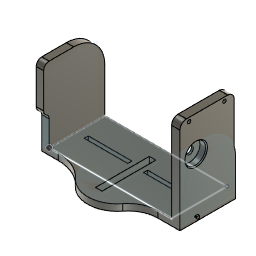
Cradle (Autodesk Fusion 360 design; units mm, degrees)
Autodesk Fusion 360 part; units mm, degrees
note: some values were not read from the file. Chosen so that the rebuilt part matches the saved one: which face or edge a step refers to; which pieces of a blend or face edit are solid. Set by a fixed rule: which sketch regions a step uses.
sketch "Szkic1" plane through (0, 0, 0) normal (0, 0, 1) x (1, 0, 0)
  line L0 (0, 0) -> (149, 0)
  line L1 (149, 0) -> (149, -85)
  line L2 (149, -85) -> (0, -85)
  line L3 (0, -85) -> (0, 0)
  line L4 (0, -85) -> (55, -85)
  line L5 (55, -85) -> (55, -60)
  line L6 (55, -60) -> (0, -60)
  line L7 (0, -60) -> (0, -85)
  line L8 (149, -85) -> (94, -85)
  line L9 (94, -85) -> (94, -60)
  line L10 (94, -60) -> (149, -60)
  line L11 (149, -60) -> (149, -85)
  dimension "d1" = 149
  dimension "d2" = 85
  dimension "d3" = 55
  dimension "d4" = 25
  dimension "d5" = 55
  dimension "d6" = 25
  constraint horizontal L0
  constraint vertical L1
  constraint horizontal L2
  constraint vertical L3
  constraint coincident L0.start L3.end
  constraint horizontal L4
  constraint vertical L5
  constraint horizontal L6
  constraint vertical L7
  constraint horizontal L8
  constraint vertical L9
  constraint horizontal L10
  constraint vertical L11
  measures "d1" distance of L0.start L0.end
  measures "d2" distance of L0.start L2.end
  measures "d3" distance of L2.end L4.end
  measures "d4" distance of L2.end L6.end
  measures "d5" distance of L1.end L8.end
  measures "d6" distance of L1.end L10.end
extrude "Wyciągnięcie proste1" add sketch "Szkic1" along normal blind 4 contours L0 L1 L2 L3 L5 L6 L9 L10
fillet "Zaokrąglenie1" radius 32 4 edges at (94, -60, 2) (94, -85, 2) (55, -85, 2) (55, -60, 2)
sketch "Szkic2" plane through (0, 0, 4) normal (0, 0, 1) x (-1, 0, 0)
  arc A0 (-49.1375, 72.4873) -> (-99.8528, 72.5) centre (-74.5, 52.9747) ccw
  arc A1 (-99.8625, 72.4873) -> (-99.8528, 72.5) centre (-125.225, 92) ccw
  arc A2 (-125.225, 60) -> (-99.8625, 72.4873) centre (-125.225, 92) ccw
  line L0 (-125.225, 60) -> (-149, 60)
  line L1 (-149, 60) -> (-149, 0)
  line L2 (-149, 0) -> (0, 0)
  line L3 (0, 0) -> (0, 60)
  line L4 (0, 60) -> (-23.775, 60)
  arc A3 (-49.1375, 72.4873) -> (-23.775, 60) centre (-23.775, 92) ccw
  line L5 (0, 0) -> (-8, 0)
  line L6 (-8, 0) -> (-8, 60)
  line L7 (-8, 60) -> (0, 60)
  line L8 (0, 60) -> (0, 0)
  line L9 (-149, 0) -> (-145, 0)
  line L10 (-145, 0) -> (-145, 60)
  line L11 (-145, 60) -> (-149, 60)
  line L12 (-149, 60) -> (-149, 0)
  constraint horizontal L5
  constraint vertical L6
  constraint horizontal L7
  constraint vertical L8
  constraint coincident L4 L6.end
  constraint coincident L2.end L3.start
  constraint horizontal L9
  constraint vertical L10
  constraint horizontal L11
  constraint vertical L12
  constraint coincident L0 L10.end
  constraint coincident L1.end L2.start
extrude "Wyciągnięcie proste2" add sketch "Szkic2" along normal blind 66 contours L2 L3 L4 L5 L6 L7 L8 | L0 L1 L2 L9 L10 L11 L12
sketch "Szkic3" plane through (0, 0, 0) normal (-1, 0, 0) x (0, -1, 0)
  line L0 (0, 0) -> (60, 0)
  line L1 (60, 0) -> (60, 70)
  line L2 (60, 70) -> (0, 70)
  line L3 (0, 70) -> (0, 0)
  circle A0 centre (42.5, 60) radius 4
  dimension "d15" = 8
  measures "d15" diameter of A0
extrude "Wyciągnięcie proste3" cut sketch "Szkic3" against normal blind 148 contours A0
extrude "Wyciągnięcie proste4" cut 1 faces at (148, -41.2702, 59.8013) along direction (1, 0, 0) blind 1
sketch "Szkic4" plane through (0, 0, 0) normal (-1, 0, 0) x (0, -1, 0)
  circle A0 centre (42.5, 60) radius 4
  line L0 (0, 0) -> (60, 0)
  line L1 (60, 0) -> (60, 70)
  line L2 (60, 70) -> (0, 70)
  line L3 (0, 70) -> (0, 0)
extrude "Wyciągnięcie proste5" add 1 faces at (5.3333, -40, 70) along direction (0, 0, 1) blind 15
sketch "Szkic5" plane through (0, -60, 0) normal (0, -1, 0) x (1, 0, 0)
  line L0 (23.775, 0) -> (23.775, 4)
  line L1 (23.775, 4) -> (8, 4)
  line L2 (8, 4) -> (8, 85)
  line L3 (8, 85) -> (0, 85)
  line L4 (0, 85) -> (0, 0)
  line L5 (0, 0) -> (23.775, 0)
  line L6 (0, 85) -> (8, 85)
  line L7 (8, 85) -> (8, 41)
  line L8 (8, 41) -> (0, 41)
  line L9 (0, 41) -> (0, 85)
  constraint horizontal L6
  constraint vertical L7
  constraint horizontal L8
  constraint vertical L9
  constraint coincident L2 L7.end
  constraint coincident L3.end L4.start
extrude "Wyciągnięcie proste6" add sketch "Szkic5" along normal blind 11 contours L2 L3 L4 L6 L7 L8 L9
sketch "Szkic6" plane through (0, 0, 0) normal (-1, 0, 0) x (0, -1, 0)
extrude "Wyciągnięcie proste7" add 1 faces at (5.3333, -63.6667, 41) along direction (0, 0, -1) blind 4
sketch "Szkic7" plane through (0, 0, 0) normal (-1, 0, 0) x (0, -1, 0)
  circle A0 centre (25.5, 77) radius 1.8
  circle A1 centre (59.5, 77) radius 1.8
  circle A2 centre (59.5, 43) radius 1.8
  circle A3 centre (25.5, 43) radius 1.8
  dimension "d28" = 3.6
  dimension "d29" = 3.6
  dimension "d30" = 3.6
  dimension "d31" = 3.6
  measures "d28" diameter of A0
  measures "d29" diameter of A1
  measures "d30" diameter of A2
  measures "d31" diameter of A3
extrude "Wyciągnięcie proste8" cut sketch "Szkic7" against normal blind 5.5
delete_face "Usuń powierzchnię1" 1 faces at (2.6667, -46.4801, 59.6017)
extrude "Wyciągnięcie proste9" cut 1 faces at (2.6667, -71, 53) along direction (0, 1, 0) blind 5
fillet "Zaokrąglenie2" radius 6 3 edges at (4, -60, 37) (4, -66, 37) (4, -66, 85)
fillet "Zaokrąglenie3" radius 33.5 2 edges at (147, 0, 70) (4, 0, 85)
sketch "Szkic8" plane through (0, 0, 4) normal (0, 0, 1) x (-1, 0, 0)
  line L0 (-145, 60) -> (-145, 0)
  line L1 (-145, 0) -> (-8, 0)
  line L2 (-8, 0) -> (-8, 60)
  line L3 (-8, 60) -> (-23.775, 60)
  arc A0 (-49.1375, 72.4873) -> (-23.775, 60) centre (-23.775, 92) ccw
  arc A1 (-49.1375, 72.4873) -> (-99.8528, 72.5) centre (-74.5, 52.9747) ccw
  arc A2 (-99.8625, 72.4873) -> (-99.8528, 72.5) centre (-125.225, 92) ccw
  arc A3 (-125.225, 60) -> (-99.8625, 72.4873) centre (-125.225, 92) ccw
  line L4 (-125.225, 60) -> (-145, 60)
  line L5 (-73, 14) -> (-80, 14)
  line L6 (-80, 14) -> (-80, 72)
  line L7 (-80, 72) -> (-73, 72)
  line L8 (-73, 72) -> (-73, 14)
  line L9 (-18, 27.8) -> (-68, 27.8)
  line L10 (-68, 27.8) -> (-68, 32.2)
  line L11 (-68, 32.2) -> (-18, 32.2)
  line L12 (-18, 32.2) -> (-18, 27.8)
  line L13 (-85, 27.8) -> (-135, 27.8)
  line L14 (-135, 27.8) -> (-135, 32.2)
  line L15 (-135, 32.2) -> (-85, 32.2)
  line L16 (-85, 32.2) -> (-85, 27.8)
  constraint horizontal L5
  constraint vertical L6
  constraint horizontal L7
  constraint vertical L8
  constraint horizontal L9
  constraint vertical L10
  constraint horizontal L11
  constraint vertical L12
  constraint horizontal L13
  constraint vertical L14
  constraint horizontal L15
  constraint vertical L16
extrude "Wyciągnięcie proste10" cut sketch "Szkic8" against normal blind 5 contours L5 L6 L7 L8 | L9 L10 L11 L12 | L13 L14 L15 L16
sketch "Szkic9" plane through (149, 0, 0) normal (1, 0, 0) x (0, 1, 0)
  arc A0 (0, 36.5) -> (-33.5, 70) centre (-33.5, 36.5) ccw
  line L0 (-33.5, 70) -> (-60, 70)
  line L1 (-60, 70) -> (-60, 0)
  line L2 (-60, 0) -> (0, 0)
  line L3 (0, 0) -> (0, 36.5)
  circle A1 centre (-42.5, 60) radius 4
  line L4 (-42.5, 60) -> (-42.5, 0)
  line L5 (-42.5, 0) -> (-41, 0)
  line L6 (-41, 0) -> (-41, 3)
  line L7 (-41, 3) -> (-42.5, 3)
  line L8 (-42.5, 3) -> (-42.5, 0)
  line L9 (-42.5, 3) -> (-44, 3)
  line L10 (-44, 3) -> (-44, 0)
  line L11 (-44, 0) -> (-42.5, 0)
  line L12 (-42.5, 0) -> (-42.5, 3)
  constraint coincident A1.centre L4.start
  constraint coincident L2 L4.end
  constraint perpendicular L2 L4
  constraint horizontal L5
  constraint vertical L6
  constraint horizontal L7
  constraint vertical L8
  constraint horizontal L9
  constraint vertical L10
  constraint horizontal L11
  constraint vertical L12
extrude "Wyciągnięcie proste11" add sketch "Szkic9" along normal blind 2 contours L2 L4 L5 L6 L7 L8 L12 | L2 L4 L8 L9 L10 L11 L12
fillet "Zaokrąglenie4" radius 2.25 1 edges at (150, -44, 0)
sketch "Szkic10" plane through (149, 0, 0) normal (1, 0, 0) x (0, 1, 0)
  line L0 (-41, 3) -> (-41, 0)
  line L1 (-41, 0) -> (0, 0)
  line L2 (0, 0) -> (0, 36.5)
  arc A0 (0, 36.5) -> (-33.5, 70) centre (-33.5, 36.5) ccw
  line L3 (-33.5, 70) -> (-60, 70)
  line L4 (-60, 70) -> (-60, 0)
  line L5 (-60, 0) -> (-41.75, 0)
  arc A1 (-44, 2.25) -> (-41.75, 0) centre (-41.75, 2.25) ccw
  line L6 (-44, 2.25) -> (-44, 3)
  line L7 (-44, 3) -> (-41, 3)
  circle A2 centre (-42.5, 60) radius 4
sketch "Szkic11" plane through (0, 0, 70) normal (0, 0, 1) x (-1, 0, 0)
  line L0 (-149, 33.5) -> (-145, 33.5)
  line L1 (-145, 33.5) -> (-145, 60)
  line L2 (-145, 60) -> (-149, 60)
  line L3 (-149, 60) -> (-149, 33.5)
delete_face "Usuń powierzchnię2" 1 faces at (33.3846, -61.477, 2.6667)
sketch "Szkic12" plane through (0, -60, 0) normal (0, -1, 0) x (1, 0, 0)
  line L0 (0, 0) -> (43.2807, 0)
  line L1 (43.2807, 0) -> (43.2807, 4)
  line L2 (43.2807, 4) -> (8, 4)
  line L3 (8, 4) -> (8, 31)
  line L4 (8, 31) -> (0, 31)
  line L5 (0, 31) -> (0, 0)
extrude "Wyciągnięcie proste13" add 1 faces at (5.3333, -42.3333, 85) along direction (0, 0, 1) blind 25
fillet "Zaokrąglenie7" radius 5 2 edges at (4, -60, 110) (4, -33.5, 110)
sketch "Szkic14" plane through (0, 0, 0) normal (-1, 0, 0) x (0, -1, 0)
  arc A0 (38.5, 110) -> (33.5, 105) centre (38.5, 105) ccw
  line L0 (33.5, 105) -> (33.5, 85)
  arc A1 (33.5, 85) -> (0, 51.5) centre (33.5, 51.5) ccw
  line L1 (0, 51.5) -> (0, 0)
  line L2 (0, 0) -> (60, 0)
  line L3 (60, 0) -> (60, 31)
  arc A2 (63, 36.1962) -> (60, 31) centre (66, 31) ccw
  arc A3 (63, 36.1962) -> (66, 41.3923) centre (60, 41.3923) ccw
  line L4 (66, 41.3923) -> (66, 79)
  arc A4 (66, 79) -> (60, 85) centre (60, 79) ccw
  line L5 (60, 85) -> (60, 105)
  arc A5 (60, 105) -> (55, 110) centre (55, 105) ccw
  line L6 (55, 110) -> (38.5, 110)
  circle A6 centre (25.5, 77) radius 1.8
  circle A7 centre (25.5, 43) radius 1.8
  circle A8 centre (59.5, 77) radius 1.8
  circle A9 centre (59.5, 43) radius 1.8
  circle A10 centre (45, 100) radius 1.8
  dimension "d63" = 3.6
  measures "d63" diameter of A10
extrude "Wyciągnięcie proste14" cut sketch "Szkic14" against normal blind 5.2 contours A10
sketch "Szkic15" plane through (8, 0, 0) normal (1, 0, 0) x (0, 1, 0)
  arc A0 (-33.5, 105) -> (-38.5, 110) centre (-38.5, 105) ccw
  line L0 (-38.5, 110) -> (-55, 110)
  arc A1 (-55, 110) -> (-60, 105) centre (-55, 105) ccw
  line L1 (-60, 105) -> (-60, 85)
  arc A2 (-60, 85) -> (-66, 79) centre (-60, 79) ccw
  line L2 (-66, 79) -> (-66, 41.3923)
  arc A3 (-66, 41.3923) -> (-63, 36.1962) centre (-60, 41.3923) ccw
  arc A4 (-60, 31) -> (-63, 36.1962) centre (-66, 31) ccw
  line L3 (-60, 31) -> (-60, 4)
  line L4 (-60, 4) -> (0, 4)
  line L5 (0, 4) -> (0, 51.5)
  arc A5 (0, 51.5) -> (-33.5, 85) centre (-33.5, 51.5) ccw
  line L6 (-33.5, 85) -> (-33.5, 105)
  circle A6 centre (-54, 104) radius 1.8
  dimension "d66" = 3.6
  measures "d66" diameter of A6
extrude "Wyciągnięcie proste15" cut sketch "Szkic15" against normal blind 5.2 contours A6
sketch "Szkic16" plane through (5.5, 0, 0) normal (-1, 0, 0) x (0, -1, 0)
  circle A0 centre (25.5, 77) radius 1.8
extrude "Wyciągnięcie proste16" add 1 faces at (145, -33.87, 32.2001) along direction (-1, 0, 0) blind 5
sketch "Szkic17" plane through (149, 0, 0) normal (1, 0, 0) x (0, 1, 0)
  circle A0 centre (-42.5, 60) radius 11
  dimension "d71" = 22
  measures "d71" diameter of A0
extrude "Wyciągnięcie proste17" add sketch "Szkic11" 1 faces at (144.6667, -42.3333, 70) along normal blind 3
extrude "Wyciągnięcie proste18" cut sketch "Szkic17" against normal blind 7
sketch "Szkic18" plane through (0, 0, 4) normal (0, 0, 1) x (-1, 0, 0)
  line L0 (-68, 27.8) -> (-68, 32.2)
  line L1 (-68, 32.2) -> (-18, 32.2)
  line L2 (-18, 32.2) -> (-18, 27.8)
  line L3 (-18, 27.8) -> (-68, 27.8)
  line L4 (-135, 27.8) -> (-135, 32.2)
  line L5 (-135, 32.2) -> (-85, 32.2)
  line L6 (-85, 32.2) -> (-85, 27.8)
  line L7 (-85, 27.8) -> (-135, 27.8)
  line L8 (-80, 14) -> (-80, 72)
  line L9 (-80, 72) -> (-73, 72)
  line L10 (-73, 72) -> (-73, 14)
  line L11 (-73, 14) -> (-80, 14)
  line L12 (-140, 60) -> (-140, 0)
  line L13 (-140, 0) -> (-8, 0)
  line L14 (-8, 0) -> (-8, 60)
  line L15 (-8, 60) -> (-43.2807, 60)
  arc A0 (-43.2807, 60) -> (-99.8625, 72.4873) centre (-74.5, 52.9747) ccw
  arc A1 (-125.225, 60) -> (-99.8625, 72.4873) centre (-125.225, 92) ccw
  line L16 (-125.225, 60) -> (-140, 60)
  line L17 (-140, 0) -> (-8, 0)
  line L18 (-8, 0) -> (-8, 60)
  line L19 (-8, 60) -> (-140, 60)
  line L20 (-140, 60) -> (-140, 0)
  constraint horizontal L17
  constraint vertical L18
  constraint horizontal L19
  constraint vertical L20
  constraint coincident L14.end L15.start
  constraint coincident L12.end L13.start
sketch "Szkic20" plane through (0, 0, 4) normal (0, 0, 1) x (-1, 0, 0)
fillet "Zaokrąglenie9" radius 45 1 edges at (43.2807, -60, 2)
sketch "Szkic21" plane through (0, 0, 4) normal (0, 0, 1) x (1, 0, 0)
extrude "Wyciągnięcie proste20" add 1 faces at (80, -33.3333, 2.6667) along direction (-1, 0, 0) blind 3
extrude "Wyciągnięcie proste21" cut 1 faces at (73, -52.6667, 2.6667) along direction (-1, 0, 0) blind 3
extrude "Wyciągnięcie proste22" add 1 faces at (68, -29.2667, 2.6667) along direction (-1, 0, 0) blind 3
extrude "Wyciągnięcie proste23" cut 1 faces at (85, -30.7333, 2.6667) along direction (-1, 0, 0) blind 3
sketch "Szkic22" plane through (0, 0, 4) normal (0, 0, 1) x (-1, 0, 0)
extrude "Wyciągnięcie proste24" add 1 faces at (146, -33.5, 71) along direction (0, 1, 0) blind 32
extrude "Wyciągnięcie proste25" add 1 faces at (143, -22.8333, 70) along direction (0, 0, -1) blind 39
extrude "Wyciągnięcie proste26" add 1 faces at (143, -40.5, 73) along direction (0, 0, 1) blind 25
sketch "Szkic23" plane through (149, 0, 0) normal (1, 0, 0) x (0, 1, 0)
  line L0 (-1.5, 46.4121) -> (-1.5, 98)
  line L1 (-1.5, 98) -> (-60, 98)
  line L2 (-60, 98) -> (-60, 0)
  line L3 (-60, 0) -> (-41.75, 0)
  arc A0 (-44, 2.25) -> (-41.75, 0) centre (-41.75, 2.25) ccw
  line L4 (-44, 2.25) -> (-44, 3)
  line L5 (-44, 3) -> (-41, 3)
  line L6 (-41, 3) -> (-41, 0)
  line L7 (-41, 0) -> (0, 0)
  line L8 (0, 0) -> (0, 36.5)
  arc A1 (0, 36.5) -> (-1.5, 46.4121) centre (-33.5, 36.5) ccw
  line L9 (-33.5, 66.3246) -> (-33.5, 53.6754)
  circle A2 centre (-42.5, 60) radius 11.16
  arc A3 (-33.5, 66.3246) -> (-33.5, 53.6754) centre (-42.5, 60) ccw
  dimension "d103" = 22.32
  measures "d103" diameter of A2
extrude "Wyciągnięcie proste27" cut sketch "Szkic23" against normal blind 7 contours L9 A3 | A2
chamfer "Fazowanie2" distance 1 angle 45 1 edges at (149, -52.9048, 64.0356)
sketch "Szkic24" plane through (149, 0, 0) normal (1, 0, 0) x (0, 1, 0)
  line L0 (-1.5, 46.4121) -> (-1.5, 98)
  line L1 (-1.5, 98) -> (-60, 98)
  line L2 (-60, 98) -> (-60, 0)
  line L3 (-60, 0) -> (-41.75, 0)
  arc A0 (-44, 2.25) -> (-41.75, 0) centre (-41.75, 2.25) ccw
  line L4 (-44, 2.25) -> (-44, 3)
  line L5 (-44, 3) -> (-41, 3)
  line L6 (-41, 3) -> (-41, 0)
  line L7 (-41, 0) -> (0, 0)
  line L8 (0, 0) -> (0, 36.5)
  arc A1 (0, 36.5) -> (-1.5, 46.4121) centre (-33.5, 36.5) ccw
  circle A2 centre (-42.5, 60) radius 12.16
  circle A3 centre (-50, 94) radius 1.8
  circle A4 centre (-12, 94) radius 1.8
  dimension "d107" = 3.6
  dimension "d108" = 3.6
  measures "d107" diameter of A3
  measures "d108" diameter of A4
fillet "Zaokrąglenie10" radius 7 2 edges at (144.5, -60, 98) (144.5, -1.5, 98)
sketch "Szkic25" plane through (0, 0, 0) normal (-1, 0, 0) x (0, -1, 0)
  circle A0 centre (45, 100) radius 1.8
  arc A1 (38.5, 110) -> (33.5, 105) centre (38.5, 105) ccw
  line L0 (33.5, 105) -> (33.5, 85)
  arc A2 (33.5, 85) -> (0, 51.5) centre (33.5, 51.5) ccw
  line L1 (0, 51.5) -> (0, 0)
  line L2 (0, 0) -> (60, 0)
  line L3 (60, 0) -> (60, 31)
  arc A3 (63, 36.1962) -> (60, 31) centre (66, 31) ccw
  arc A4 (63, 36.1962) -> (66, 41.3923) centre (60, 41.3923) ccw
  line L4 (66, 41.3923) -> (66, 79)
  arc A5 (66, 79) -> (60, 85) centre (60, 79) ccw
  line L5 (60, 85) -> (60, 105)
  arc A6 (60, 105) -> (55, 110) centre (55, 105) ccw
  line L6 (55, 110) -> (38.5, 110)
  circle A7 centre (25.5, 77) radius 1.8
  circle A8 centre (25.5, 43) radius 1.8
  circle A9 centre (59.5, 77) radius 1.8
  circle A10 centre (59.5, 43) radius 1.8
  line L7 (33.5, 85) -> (60, 85)
  line L8 (60, 85) -> (60, 110)
  line L9 (60, 110) -> (33.5, 110)
  line L10 (33.5, 110) -> (33.5, 85)
  constraint horizontal L7
  constraint vertical L8
  constraint horizontal L9
  constraint vertical L10
  constraint coincident L0.end A2.start
extrude "Wyciągnięcie proste28" cut sketch "Szkic25" against normal blind 10 contours A0 | A1 L0 L5 A6 L6 L7 L8 L9 L10
extrude "Wyciągnięcie proste29" cut sketch "Szkic24" against normal blind 5.5 contours A3 | A4
sketch "Szkic26" plane through (0, 0, 0) normal (0, 0, -1) x (1, 0, 0)
  line L0 (17.7341, 60) -> (0, 60)
  line L1 (0, 60) -> (0, 0)
  line L2 (0, 0) -> (149, 0)
  line L3 (149, 0) -> (149, 41)
  line L4 (149, 41) -> (151, 41)
  line L5 (151, 41) -> (151, 41.75)
  line L6 (151, 41.75) -> (149, 41.75)
  line L7 (149, 41.75) -> (149, 60)
  line L8 (149, 60) -> (125.225, 60)
  arc A0 (99.8625, 72.4873) -> (125.225, 60) centre (125.225, 92) ccw
  arc A1 (99.8625, 72.4873) -> (50.909, 74.5956) centre (74.5, 52.9747) ccw
  arc A2 (17.7341, 60) -> (50.909, 74.5956) centre (17.7341, 105) ccw
  line L9 (65, 27.8) -> (18, 27.8)
  line L10 (18, 27.8) -> (18, 32.2)
  line L11 (18, 32.2) -> (65, 32.2)
  line L12 (65, 32.2) -> (65, 27.8)
  line L13 (135, 27.8) -> (82, 27.8)
  line L14 (82, 27.8) -> (82, 32.2)
  line L15 (82, 32.2) -> (135, 32.2)
  line L16 (135, 32.2) -> (135, 27.8)
  line L17 (77, 14) -> (70, 14)
  line L18 (70, 14) -> (70, 72)
  line L19 (70, 72) -> (77, 72)
  line L20 (77, 72) -> (77, 14)
  line L21 (149, 41) -> (149, 41.75)
  constraint coincident L3.end L4.start
  constraint coincident L6.end L7.start
extrude "Wyciągnięcie proste30" add sketch "Szkic26" along normal blind 3 contours L0 L1 L2 L3 L7 L8 A0 A1 A2 L21
